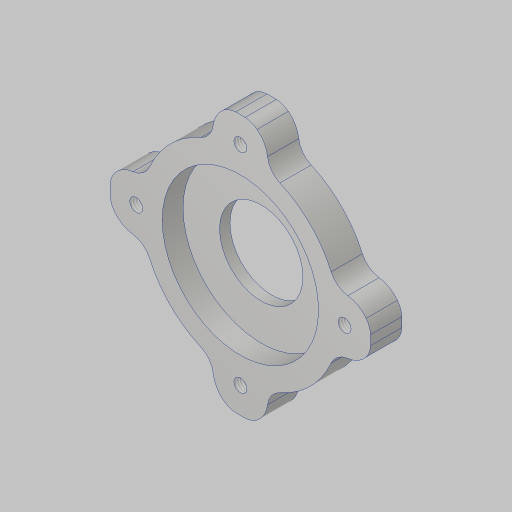
# Autodesk Inventor part: CL7-013
Saved by Autodesk Inventor 2023.5 (Build 275446000, 446)
## iProperties
Created: 2025-03-18
Part Number: CL7-013
Material: Aluminum 6061
Document SubType Name: Modeling
Designer: brand
Density: 2.7 g/cm^3
Appearance: Aluminum - Flat
Author: brand
Autodesk Inventor part; units mm, degrees
ref_plane "YZ Plane" through (0, 0, 0) normal (1, 0, 0) x (0, 1, 0)
ref_plane "XZ Plane" through (0, 0, 0) normal (0, 1, 0) x (-1, 0, 0)
ref_plane "XY Plane" through (0, 0, 0) normal (0, 0, 1) x (1, 0, 0)
sketch "Sketch1" plane through (0, 0, 0) normal (0, 0, 1) x (1, 0, 0)
  circle A0 centre (0, 0) radius 23.8125
  circle A1 centre (0, 0) radius 39.6875
  circle A2 centre (0, 0) radius 31.75 construction
  circle A3 centre (0, 0) radius 12.7
  point P0 (0, 31.75)
  point P1 (-31.75, 0)
  point P2 (31.75, 0)
  point P3 (0, -31.75)
  dimension "d0" = 47.625
  dimension "d1" = 15.875
  dimension "d2" = 63.5
  dimension "d5" = 25.4
  constraints: 4 centre point, 4 point on circle, 3 coincident, 2 horizontal alignment, 2 vertical alignment
  measures "d0" diameter of A0
  measures "d1" radial gap between concentric circles of A0 A1
  measures "d2" diameter of A2
  measures "d5" diameter of A3
extrude "Extrusion1" add sketch "Sketch1" against normal blind 9.525 contours A0 | A1
extrude "Extrusion2" cut sketch "Sketch1" against normal blind 6.35 contours A0
hole "Hole1" at (0, 31.75, 0) at (-31.75, 0, 0) at (31.75, 0, 0) at (0, -31.75, 0) direction (0, 0, -1) diameter 3.9624 end through all thread size "10-32 UNF" class "2B" standard "ANSI Unified Screw Threads"
sketch "Sketch2" plane through (0, 0, 0) normal (0, 0, 1) x (1, 0, 0)
  circle A0 centre (31.75, 0) radius 1.9812 construction
  circle A1 centre (0, 31.75) radius 1.9812 construction
  circle A2 centre (-31.75, 0) radius 1.9812 construction
  circle A3 centre (0, -31.75) radius 1.9812 construction
  circle A4 centre (0, 0) radius 23.8125 construction
  circle A5 centre (0, 0) radius 39.6875 construction
  circle A6 centre (0, 31.75) radius 8.3312 construction
  circle A7 centre (31.75, 0) radius 8.3312 construction
  circle A8 centre (0, 0) radius 30.1625 construction
  circle A9 centre (-31.75, 0) radius 8.3312 construction
  circle A10 centre (0, -31.75) radius 8.3312 construction
  arc A11 (-27.6536, -12.0439) -> (-32.7291, -8.2735) centre (-33.4754, -14.5795) ccw
  line L0 (0, 0) -> (-28.0633, -28.0633) construction
  line L1 (0, 0) -> (-31.75, 0) construction
  circle A12 centre (0, 0) radius 39.6875 construction
  arc A13 (-39.5866, -2.8277) -> (-32.7291, -8.2735) centre (-31.75, 0) ccw
  arc A14 (-27.6536, -12.0439) -> (-12.0439, -27.6536) centre (0, 0) ccw
  arc A15 (-8.2735, -32.7291) -> (-12.0439, -27.6536) centre (-14.5795, -33.4754) ccw
  line L2 (-33.4754, -14.5795) -> (-14.5795, -33.4754) construction
  circle A16 centre (-31.75, 0) radius 1.9812 construction
  line L3 (0, 0) -> (-31.75, 0) construction
  line L4 (0, 0) -> (0, -31.75) construction
  arc A17 (-8.2735, -32.7291) -> (-2.8277, -39.5866) centre (0, -31.75) ccw
  arc A18 (-32.7291, 8.2735) -> (-27.6536, 12.0439) centre (-33.4754, 14.5795) ccw
  arc A19 (-32.7291, 8.2735) -> (-39.5866, 2.8277) centre (-31.75, 0) ccw
  arc A20 (-12.0439, 27.6536) -> (-27.6536, 12.0439) centre (0, 0) ccw
  arc A21 (-12.0439, 27.6536) -> (-8.2735, 32.7291) centre (-14.5795, 33.4754) ccw
  arc A22 (-2.8277, 39.5866) -> (-8.2735, 32.7291) centre (0, 31.75) ccw
  arc A23 (-39.5866, 2.8277) -> (-39.5866, -2.8277) centre (0, 0) ccw construction
  line L5 (0, 0) -> (28.0633, -28.0633) construction
  circle A24 centre (0, 0) radius 39.6875 construction
  circle A25 centre (0, 0) radius 39.6875
  arc A26 (32.7291, -8.2735) -> (27.6536, -12.0439) centre (33.4754, -14.5795) ccw
  arc A27 (18.464, -23.8507) -> (27.6536, -12.0439) centre (0, 0) ccw
  arc A28 (2.8277, -39.5866) -> (6.9771, -36.303) centre (0, -31.75) ccw
  arc A29 (32.7291, -8.2735) -> (39.5866, -2.8277) centre (31.75, 0) ccw
  point P0 (-2.8277, 39.5866)
  point P1 (-39.5866, 2.8277)
  point P2 (-2.8277, -39.5866)
  dimension "d15" = 6.35
  dimension "d16" = 6.35
  dimension "d17" = 6.35
  dimension "d18" = 6.35
  dimension "d19" = 6.35
  dimension "d20" = 45
  dimension "d21" = 6.35
  dimension "d22" = 45
  dimension "d27" = 6.35
  constraints: 42 point on circle, 20 centre point, 14 symmetric about line, 12 end point, 7 coincident, 5 tangent, 3 concentric, 2 horizontal, 2 point on line, 1 vertical, 13 other
  measures "d15" radial gap between concentric circles of A1 A6
  measures "d16" radial gap between concentric circles of A0 A7
  measures "d17" radial gap between concentric circles of A4 A8
  measures "d18" radial gap between concentric circles of A2 A9
  measures "d19" radial gap between concentric circles of A3 A10
  measures "d20" angle of L0 L1
  measures "d21" radius of A11
  measures "d22" angle of L5 L4
  measures "d27" radius of A26
extrude "Extrusion3" cut sketch "Sketch2" against normal through all contours A14 A15 A17 A25 A13 A11 | A25 A22 A21 A20 A18 A19
mirror "Mirror1" about plane through (0, 0, 0) normal (1, 0, 0) of "Extrusion3"
fillet "Fillet1" radius 6.35 8 edges at (-39.5866, 2.8277, -4.7625) (-39.5866, -2.8277, -4.7625) (2.8277, 39.5866, -4.7625) (-2.8277, 39.5866, -4.7625) (39.5866, 2.8277, -4.7625) (39.5866, -2.8277, -4.7625) (2.8277, -39.5866, -4.7625) (-2.8277, -39.5866, -4.7625)
equation "\"d22\" = d20"
equation "\"d27\" = d26"
equation "\"d26\" = d21"
body "Solid1"
